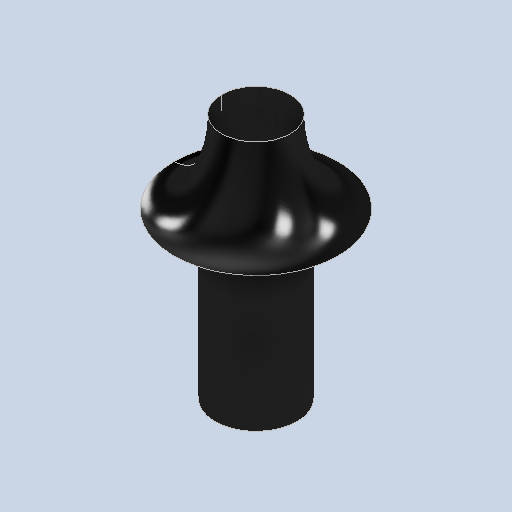
# Autodesk Inventor part: TorsOsc-2025-Cell-CapGlue
Saved by Autodesk Inventor 2026 (Build 300175050, 175E)
## iProperties
Created: 2023-08-21
Part Number: TorsOsc-2025-Cell-CapGlue
Material: Polycarbonate, Smoke
Document SubType Name: Modeling
Designer: schanen
Density: 1.2 g/cm^3
Appearance: Black
Author: schanen
Autodesk Inventor part; units mm, degrees
ref_plane "YZ Plane" through (0, 0, 0) normal (1, 0, 0) x (0, 1, 0)
ref_plane "XZ Plane" through (0, 0, 0) normal (0, 1, 0) x (-1, 0, 0)
ref_plane "XY Plane" through (0, 0, 0) normal (0, 0, 1) x (1, 0, 0)
sketch "Sketch1" plane through (0, 0, 0) normal (0, 0, 1) x (1, 0, 0)
  line L0 (-0.625, 0) -> (-0.625, 1.5)
  line L1 (-0.625, 0) -> (-1.5, 0)
  ellipse E0 centre (-1.5, 1.5) end of major axis (-1.5, 0) minor radius 0.875
  line L2 (0, -0.6) -> (0, 3.6) projected
  point P0 (0, 0)
  dimension "d0" = 1.5
  dimension "d1" = 0.625
  dimension "d2" = 1.5
  constraints: 4 end point, 1 horizontal, 1 horizontal alignment, 1 vertical, 1 vertical alignment, 4 other
  measures "d0" distance of point (0, 0) L1.end
  measures "d1" distance from line of point (0, 0) L0
  measures "d2" distance of L0.start L0.end
revolve "Revolution1" add sketch "Sketch1" angle 360 about axis through (0, -10, 0) along (0, 1, 0) contours L1 E0 L0
sketch "Sketch2" plane through (0, 0, 0) normal (0, -1, 0) x (1, 0, 0)
  circle A0 centre (0, 0) radius 0.75
  circle A1 centre (0, 0) radius 0.625
  circle A2 centre (0, 0) radius 0.625 projected
  dimension "d4" = 1.5
  constraints: 2 centre point, 2 coincident, 1 concentric
  measures "d4" diameter of A0
extrude "Extrusion1" add sketch "Sketch2" along normal blind 3
body "Solid1"
